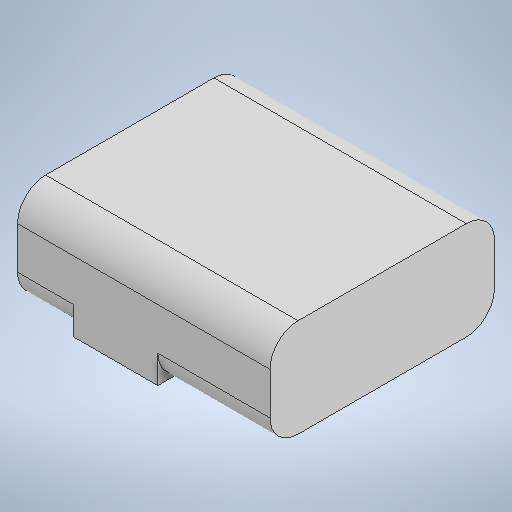
# Autodesk Inventor part: USB-C
Saved by Autodesk Inventor 2025.2 (Build 292293000, 293)
## iProperties
Created: 2024-11-18
Part Number: USB-C
Material: Generisch
Document SubType Name: Modeling
Designer: tills
Density: 1 g/cm^3
Appearance: Vorgabe
Author: tills
Autodesk Inventor part; units mm, degrees
ref_plane "YZ Plane" through (0, 0, 0) normal (1, 0, 0) x (0, 1, 0)
ref_plane "XZ Plane" through (0, 0, 0) normal (0, 1, 0) x (-1, 0, 0)
ref_plane "XY Plane" through (0, 0, 0) normal (0, 0, 1) x (1, 0, 0)
sketch "Skizze1" plane through (0, 0, 0) normal (0, 1, 0) x (-1, 0, 0)
  line L0 (4.5, 4) -> (-4.5, 4)
  line L1 (-4.5, 4) -> (-4.5, -4)
  line L2 (-4.5, -4) -> (4.5, -4)
  line L3 (4.5, -4) -> (4.5, 4)
  line L4 (4.5, 4) -> (-4.5, -4) construction
  line L5 (-4.5, 4) -> (4.5, -4) construction
  point P0 (0, 0)
  dimension "d0" = 9
  dimension "d1" = 8
  constraints: 12 end point, 2 midpoint, 2 parallel, 1 horizontal, 1 perpendicular
  measures "d0" distance of L1.end L2.end
  measures "d1" distance of L0.end L1.end
extrude "Extrusion1" add sketch "Skizze1" along normal blind 3.5
fillet "Rundung1" radius 1 4 edges at (0, 3.5, 4) (0, 0, 4) (0, 3.5, -4) (0, 0, -4)
sketch "Skizze2" plane through (-4.5, 0, -3) normal (-1, 0, 0) x (0, 0, 1)
  line L0 (-1, 1) -> (-1, 2.5) projected
  arc A0 (0, 3.5) -> (-1, 2.5) centre (0, 2.5) ccw projected
  line L1 (0, 3.5) -> (6, 3.5) projected
  arc A1 (7, 2.5) -> (6, 3.5) centre (6, 2.5) ccw projected
  line L2 (7, 1) -> (7, 2.5) projected
  arc A2 (6, 0) -> (7, 1) centre (6, 1) ccw projected
  line L3 (0, 0) -> (6, 0) projected
  arc A3 (-1, 1) -> (0, 0) centre (0, 1) ccw projected
  line L4 (0.5, 2.5) -> (5.5, 2.5)
  line L5 (6, 2) -> (6, 1.5)
  line L6 (5.5, 1) -> (0.5, 1)
  line L7 (0, 1.5) -> (0, 2)
  arc A4 (0.5, 2.5) -> (0, 2) centre (0.5, 2) ccw
  arc A5 (0, 1.5) -> (0.5, 1) centre (0.5, 1.5) ccw
  arc A6 (5.5, 1) -> (6, 1.5) centre (5.5, 1.5) ccw
  arc A7 (6, 2) -> (5.5, 2.5) centre (5.5, 2) ccw
  line L8 (0, 3.1) -> (6, 3.1)
  line L9 (0, 0.4) -> (6, 0.4)
  line L10 (-0.6, 2.5) -> (-0.6, 1)
  line L11 (6.6, 2.5) -> (6.6, 1)
  arc A8 (0, 3.1) -> (-0.6, 2.5) centre (0, 2.5) ccw
  arc A9 (6.6, 2.5) -> (6, 3.1) centre (6, 2.5) ccw
  arc A10 (6, 0.4) -> (6.6, 1) centre (6, 1) ccw
  arc A11 (-0.6, 1) -> (0, 0.4) centre (0, 1) ccw
  point P0 (3, 0)
  dimension "d5" = 0.5
  dimension "d6" = 0.4
  dimension "d7" = 0.4
  dimension "d8" = 0.4
  dimension "d9" = 0.4
  constraints: 16 end point, 16 point on circle, 12 tangent, 8 centre point, 4 point on line, 3 equal radius, 3 horizontal, 2 parallel, 2 vertical, 1 perpendicular
  measures "d5" radius of A4
  measures "d6" distance between parallel lines of L1 L8
  measures "d7" distance between parallel lines of L3 L9
  measures "d8" distance between parallel lines of L2 L11
  measures "d9" distance between parallel lines of L0 L10
extrude "Extrusion2" cut sketch "Skizze2" against normal blind 5 contours L8 A9 L11 A10 L9 A11 L10 A8
sketch "Skizze3" plane through (0, 0, 0) normal (0, -1, 0) x (1, 0, 0)
  line L0 (-4.5, 3) -> (4.5, 3) projected
  line L1 (4.5, 4) -> (-4.5, 4) projected
  line L2 (-2.5, 3) -> (0.5, 3)
  line L3 (0.5, 3) -> (0.5, 4)
  line L4 (0.5, 4) -> (-2.5, 4)
  line L5 (-2.5, 4) -> (-2.5, 3)
  line L6 (-4.5, 3) -> (-4.5, 4) projected
  line L7 (-2.8823, 0) -> (1.7829, 0)
  line L8 (-4.5, -3) -> (4.5, -3)
  line L9 (4.5, -4) -> (-4.5, -4)
  line L10 (0.5, -3) -> (0.5, -4)
  line L11 (-2.5, -4) -> (-2.5, -3)
  point P0 (0, 0)
  dimension "d12" = 2
  dimension "d13" = 3
  constraints: 18 end point, 8 symmetric about line, 4 point on line, 2 horizontal, 2 parallel, 1 perpendicular
  measures "d12" distance between parallel lines of L6 L5
  measures "d13" distance between parallel lines of L3 L5
extrude "Extrusion3" add sketch "Skizze3" against normal blind 1 contours L5 L1 L3 L0 | L8 L10 L9 L11
